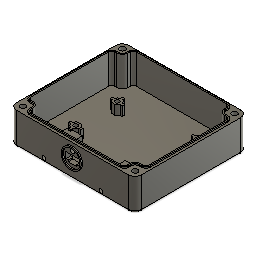
RPLIDAR Enclosure Base v7 (Autodesk Fusion 360 design; units mm, degrees)
Autodesk Fusion 360 part; units mm, degrees
sketch "Sketch1" plane through (0, 0, 0) normal (0, 1, 0) x (1, 0, 0)
  line L0 (6.35, 0) -> (110.49, 0)
  line L1 (116.84, 6.35) -> (116.84, 72.0491)
  line L2 (0, 72.0491) -> (0, 6.35)
  arc A0 (0, 6.35) -> (6.35, 0) centre (6.35, 6.35) ccw
  arc A1 (110.49, 0) -> (116.84, 6.35) centre (110.49, 6.35) ccw
  arc A2 (112.9511, 77.9028) -> (58.42, 88.9) centre (58.42, -51.7982) ccw
  arc A3 (58.42, 88.9) -> (3.8889, 77.9027) centre (58.42, -51.7979) ccw
  arc A4 (3.8889, 77.9027) -> (0, 72.0491) centre (6.35, 72.0491) ccw
  arc A5 (116.84, 72.0491) -> (112.9511, 77.9028) centre (110.49, 72.0491) ccw
  line L3 (2.286, 72.0491) -> (2.286, 6.35)
  arc A6 (2.286, 6.35) -> (6.35, 2.286) centre (6.35, 6.35) ccw
  line L4 (6.35, 2.286) -> (110.49, 2.286)
  arc A7 (110.49, 2.286) -> (114.554, 6.35) centre (110.49, 6.35) ccw
  line L5 (114.554, 6.35) -> (114.554, 72.0491)
  arc A8 (114.554, 72.0491) -> (112.0651, 75.7954) centre (110.49, 72.0491) ccw
  arc A9 (112.0651, 75.7954) -> (58.42, 86.614) centre (58.42, -51.7982) ccw
  arc A10 (58.42, 86.614) -> (4.7749, 75.7954) centre (58.42, -51.7979) ccw
  arc A11 (4.7749, 75.7954) -> (2.286, 72.0491) centre (6.35, 72.0491) ccw
  point P0 (116.84, 0)
  dimension "d1" = 116.84
  dimension "d3" = 6.35
  dimension "d4" = 6.35
  dimension "d5" = 6.35
  dimension "d6" = 6.35
  dimension "d7" = 2.286
  constraint horizontal L0
  constraint vertical L1
  constraint vertical L2
  constraint coincident origin L0
  constraint coincident origin L2
  constraint tangent L0 A0
  constraint tangent L2 A0
  constraint coincident P0 L0
  constraint coincident P0 L1
  constraint tangent L0 A1
  constraint tangent L1 A1
  constraint tangent A3 A4
  constraint tangent L2 A4
  constraint tangent A2 A5
  constraint tangent L1 A5
  measures "d1" distance of origin P0
  measures "d3" radius of A0
  measures "d4" radius of A1
  measures "d5" radius of A4
  measures "d6" radius of A5
mesh "Mesh1" [no effect]
sketch "Sketch2" plane through (0, 0, 0) normal (0, 1, 0) x (-1, 0, 0)
  line L0 (-23.4602, -26.5297) -> (-24.9674, -28.9918)
  line L1 (-24.9674, -28.9918) -> (-27.8532, -28.9176)
  line L2 (-27.8532, -28.9176) -> (-29.2318, -26.3814)
  line L3 (-29.2318, -26.3814) -> (-27.7247, -23.9193)
  line L4 (-27.7247, -23.9193) -> (-24.8389, -23.9934)
  line L5 (-24.8389, -23.9934) -> (-23.4602, -26.5297)
  circle A0 centre (-22.846, -46.4555) radius 15.9986
  circle A1 centre (-26.3276, -66.4551) radius 2.7647
  circle A2 centre (-26.3276, -26.456) radius 2.7647
  circle A3 centre (-96.3501, -74.4876) radius 2.7745
  circle A4 centre (-96.3712, -18.4353) radius 2.7744
sketch "Sketch3" plane through (0, 0, 0) normal (0, 1, 0) x (1, 0, 0)
  line L0 (13.5354, -5.4011) -> (100.9114, -5.4011)
  line L1 (115.3275, 9.026) -> (115.1243, 84.21)
  line L2 (100.9114, 98.6151) -> (13.5354, 98.6151)
  line L3 (-0.8807, 84.188) -> (-0.6775, 9.004)
  line L4 (104.9754, -1.3371) -> (104.9754, 0.887)
  line L5 (109.0394, 4.951) -> (111.2635, 4.951)
  line L6 (9.4714, -1.3371) -> (9.4714, 0.887)
  line L7 (5.4074, 4.951) -> (3.3865, 4.951)
  line L8 (104.9754, 94.5511) -> (104.9754, 92.327)
  line L9 (109.0394, 88.263) -> (111.0603, 88.263)
  line L10 (9.4714, 94.5511) -> (9.4714, 92.327)
  line L11 (5.4074, 88.263) -> (3.1833, 88.263)
  circle A0 centre (3.2484, 94.486) radius 2.9718
  circle A1 centre (111.1984, 94.486) radius 2.9718
  circle A2 centre (111.1984, -1.27) radius 2.9718
  circle A3 centre (3.2484, -1.27) radius 2.9718
  arc A4 (104.9754, 94.5511) -> (100.9114, 98.6151) centre (100.9114, 94.5511) ccw
  arc A5 (115.1243, 84.21) -> (111.0603, 88.263) centre (111.0603, 84.199) ccw
  arc A6 (104.9754, 92.327) -> (109.0394, 88.263) centre (109.0394, 92.327) ccw
  arc A7 (111.2635, 4.951) -> (115.3275, 9.026) centre (111.2635, 9.015) ccw
  arc A8 (100.9114, -5.4011) -> (104.9754, -1.3371) centre (100.9114, -1.3371) ccw
  arc A9 (109.0394, 4.951) -> (104.9754, 0.887) centre (109.0394, 0.887) ccw
  line L12 (3.4676, -7.7324) -> (111.1636, -7.7324)
  line L13 (117.5136, -1.3824) -> (117.5136, 94.1216)
  line L14 (111.1636, 100.4716) -> (3.4676, 100.4716)
  line L15 (-2.8824, 94.1216) -> (-2.8824, -1.3824)
  arc A10 (3.4676, 100.4716) -> (-2.8824, 94.1216) centre (3.4676, 94.1216) ccw
  arc A11 (117.5136, 94.1216) -> (111.1636, 100.4716) centre (111.1636, 94.1216) ccw
  arc A12 (111.1636, -7.7324) -> (117.5136, -1.3824) centre (111.1636, -1.3824) ccw
  arc A13 (-2.8824, -1.3824) -> (3.4676, -7.7324) centre (3.4676, -1.3824) ccw
  arc A14 (13.5354, 98.6151) -> (9.4714, 94.5511) centre (13.5354, 94.5511) ccw
  arc A15 (3.1833, 88.263) -> (-0.8807, 84.188) centre (3.1833, 84.199) ccw
  arc A16 (-0.6775, 9.004) -> (3.3865, 4.951) centre (3.3865, 9.015) ccw
  arc A17 (9.4714, -1.3371) -> (13.5354, -5.4011) centre (13.5354, -1.3371) ccw
  arc A18 (9.4714, 0.887) -> (5.4074, 4.951) centre (5.4074, 0.887) ccw
  arc A19 (5.4074, 88.263) -> (9.4714, 92.327) centre (5.4074, 92.327) ccw
  circle A20 centre (96.3501, 74.4876) radius 2.0193
  circle A21 centre (96.3712, 18.4353) radius 2.0193
  circle A22 centre (26.3276, 26.456) radius 2.0193
  circle A23 centre (26.3276, 66.4551) radius 2.0193
  arc A24 (27.2538, 62.498) -> (24.1187, 63.0438) centre (22.846, 46.4555) ccw
  arc A25 (24.1186, 29.8673) -> (27.2538, 30.413) centre (22.846, 46.4555) ccw
  line L16 (90.3811, 73.4716) -> (90.3811, 75.5036)
  line L17 (102.3191, 75.5036) -> (102.3191, 73.4716)
  line L18 (102.3191, 73.4716) -> (90.3811, 75.5036) construction
  line L19 (90.3811, 73.4716) -> (102.3191, 75.5036) construction
  line L20 (97.3661, 80.4566) -> (95.3341, 80.4566)
  line L21 (95.3341, 68.5186) -> (97.3661, 68.5186)
  line L22 (97.3661, 80.4566) -> (95.3341, 68.5186) construction
  line L23 (95.3341, 80.4566) -> (97.3661, 68.5186) construction
  line L24 (95.3341, 80.4566) -> (95.3341, 78.4226)
  line L25 (95.3341, 70.5527) -> (95.3341, 68.5186)
  line L26 (97.3661, 68.5186) -> (97.3661, 70.5527)
  line L27 (97.3661, 78.4226) -> (97.3661, 80.4566)
  arc A26 (97.3661, 70.5527) -> (100.2851, 73.4716) centre (96.3501, 74.4876) ccw
  arc A27 (100.2851, 75.5036) -> (97.3661, 78.4226) centre (96.3501, 74.4876) ccw
  line L28 (102.3191, 73.4716) -> (100.2851, 73.4716)
  line L29 (92.4152, 73.4716) -> (90.3811, 73.4716)
  arc A28 (95.3341, 78.4226) -> (92.4152, 75.5036) centre (96.3501, 74.4876) ccw
  arc A29 (92.4152, 73.4716) -> (95.3341, 70.5527) centre (96.3501, 74.4876) ccw
  line L30 (90.3811, 75.5036) -> (92.4152, 75.5036)
  line L31 (100.2851, 75.5036) -> (102.3191, 75.5036)
  line L32 (97.3872, 24.4043) -> (95.3552, 24.4043)
  line L33 (95.3552, 12.4663) -> (97.3872, 12.4663)
  line L34 (97.3872, 24.4043) -> (95.3552, 12.4663) construction
  line L35 (95.3552, 24.4043) -> (97.3872, 12.4663) construction
  line L36 (90.4022, 19.4513) -> (90.4022, 17.4193)
  line L37 (102.3402, 17.4193) -> (102.3402, 19.4513)
  line L38 (102.3402, 19.4513) -> (90.4022, 17.4193) construction
  line L39 (90.4022, 19.4513) -> (102.3402, 17.4193) construction
  line L40 (97.3872, 12.4663) -> (97.3872, 14.5004)
  line L41 (97.3872, 22.3703) -> (97.3872, 24.4043)
  line L42 (95.3552, 24.4043) -> (95.3552, 22.3703)
  line L43 (95.3552, 14.5004) -> (95.3552, 12.4663)
  arc A30 (97.3872, 14.5004) -> (100.3061, 17.4193) centre (96.3712, 18.4353) ccw
  arc A31 (100.3061, 19.4513) -> (97.3872, 22.3703) centre (96.3712, 18.4353) ccw
  line L44 (90.4022, 17.4193) -> (92.4362, 17.4193)
  line L45 (100.3061, 17.4193) -> (102.3402, 17.4193)
  arc A32 (95.3552, 22.3703) -> (92.4362, 19.4513) centre (96.3712, 18.4353) ccw
  arc A33 (92.4362, 17.4193) -> (95.3552, 14.5004) centre (96.3712, 18.4353) ccw
  line L46 (102.3402, 19.4513) -> (100.3061, 19.4513)
  line L47 (92.4362, 19.4513) -> (90.4022, 19.4513)
  line L48 (20.3586, 25.44) -> (20.3586, 27.472)
  line L49 (32.2966, 27.472) -> (32.2966, 25.44)
  line L50 (32.2966, 25.44) -> (20.3586, 27.472) construction
  line L51 (20.3586, 25.44) -> (32.2966, 27.472) construction
  line L52 (20.3586, 27.472) -> (22.3926, 27.472)
  line L53 (30.2625, 27.472) -> (32.2966, 27.472)
  arc A34 (30.2625, 27.472) -> (27.2538, 30.413) centre (26.3276, 26.456) ccw
  line L54 (32.2966, 25.44) -> (30.2625, 25.44)
  line L55 (22.3926, 25.44) -> (20.3586, 25.44)
  arc A35 (24.1186, 29.8673) -> (22.3926, 27.472) centre (26.3276, 26.456) ccw
  line L56 (27.3436, 20.487) -> (25.3116, 20.487)
  line L57 (27.3436, 22.5211) -> (27.3436, 20.487)
  line L58 (27.3436, 20.487) -> (25.3116, 32.425) construction
  line L59 (25.3116, 20.487) -> (27.3436, 32.425) construction
  arc A36 (22.3926, 25.44) -> (25.3116, 22.5211) centre (26.3276, 26.456) ccw
  arc A37 (27.3436, 22.5211) -> (30.2625, 25.44) centre (26.3276, 26.456) ccw
  line L60 (25.3116, 20.487) -> (25.3116, 22.5211)
  line L61 (20.3586, 67.4711) -> (20.3586, 65.4391)
  line L62 (32.2966, 65.4391) -> (32.2966, 67.4711)
  line L63 (32.2966, 67.4711) -> (20.3586, 65.4391) construction
  line L64 (20.3586, 67.4711) -> (32.2966, 65.4391) construction
  arc A38 (22.3926, 65.4391) -> (24.1187, 63.0438) centre (26.3276, 66.4551) ccw
  line L65 (32.2966, 67.4711) -> (30.2625, 67.4711)
  line L66 (22.3926, 67.4711) -> (20.3586, 67.4711)
  line L67 (20.3586, 65.4391) -> (22.3926, 65.4391)
  line L68 (30.2625, 65.4391) -> (32.2966, 65.4391)
  arc A39 (27.2538, 62.498) -> (30.2625, 65.4391) centre (26.3276, 66.4551) ccw
  line L69 (27.3436, 72.4241) -> (25.3116, 72.4241)
  line L70 (27.3436, 72.4241) -> (25.3116, 60.4861) construction
  line L71 (25.3116, 72.4241) -> (27.3436, 60.4861) construction
  arc A40 (30.2625, 67.4711) -> (27.3436, 70.39) centre (26.3276, 66.4551) ccw
  arc A41 (25.3116, 70.39) -> (22.3926, 67.4711) centre (26.3276, 66.4551) ccw
  line L72 (25.3116, 72.4241) -> (25.3116, 70.39)
  line L73 (27.3436, 70.39) -> (27.3436, 72.4241)
  line L74 (5.4074, 6.1702) -> (3.3865, 6.1702)
  arc A42 (0.5417, 9.0073) -> (3.3865, 6.1702) centre (3.3865, 9.015) ccw
  line L75 (0.3385, 84.1913) -> (0.5417, 9.0073)
  arc A43 (3.1833, 87.0438) -> (0.3385, 84.1913) centre (3.1833, 84.199) ccw
  line L76 (5.4074, 87.0438) -> (3.1833, 87.0438)
  arc A44 (5.4074, 87.0438) -> (10.6906, 92.327) centre (5.4074, 92.327) ccw
  line L77 (10.6906, 94.5511) -> (10.6906, 92.327)
  arc A45 (13.5354, 97.3959) -> (10.6906, 94.5511) centre (13.5354, 94.5511) ccw
  line L78 (100.9114, 97.3959) -> (13.5354, 97.3959)
  arc A46 (103.7562, 94.5511) -> (100.9114, 97.3959) centre (100.9114, 94.5511) ccw
  line L79 (103.7562, 94.5511) -> (103.7562, 92.327)
  arc A47 (103.7562, 92.327) -> (109.0394, 87.0438) centre (109.0394, 92.327) ccw
  line L80 (109.0394, 87.0438) -> (111.0603, 87.0438)
  arc A48 (113.9051, 84.2067) -> (111.0603, 87.0438) centre (111.0603, 84.199) ccw
  line L81 (114.1083, 9.0227) -> (113.9051, 84.2067)
  arc A49 (111.2635, 6.1702) -> (114.1083, 9.0227) centre (111.2635, 9.015) ccw
  line L82 (109.0394, 6.1702) -> (111.2635, 6.1702)
  arc A50 (109.0394, 6.1702) -> (103.7562, 0.887) centre (109.0394, 0.887) ccw
  line L83 (103.7562, -1.3371) -> (103.7562, 0.887)
  arc A51 (100.9114, -4.1819) -> (103.7562, -1.3371) centre (100.9114, -1.3371) ccw
  line L84 (13.5354, -4.1819) -> (100.9114, -4.1819)
  arc A52 (10.6906, -1.3371) -> (13.5354, -4.1819) centre (13.5354, -1.3371) ccw
  line L85 (10.6906, -1.3371) -> (10.6906, 0.887)
  arc A53 (10.6906, 0.887) -> (5.4074, 6.1702) centre (5.4074, 0.887) ccw
  line L86 (14.265, -3.1639) -> (101.4284, -3.1639)
  arc A54 (10.6906, -0.3368) -> (14.265, -3.1639) centre (14.265, 0.5093) ccw
  arc A55 (101.4284, -3.1639) -> (103.7562, -1.3426) centre (101.4284, -0.7657) ccw
  line L87 (23.0256, -7.7324) -> (36.7416, -7.7324)
  line L88 (36.7416, -7.7324) -> (36.7416, 22.4936)
  line L89 (36.7416, 22.4936) -> (23.0256, 22.4936)
  line L90 (23.0256, 22.4936) -> (23.0256, -7.7324)
  line L91 (91.6056, -7.7324) -> (77.8896, -7.7324)
  line L92 (77.8896, -7.7324) -> (77.8896, 22.4936)
  line L93 (77.8896, 22.4936) -> (91.6056, 22.4936)
  line L94 (91.6056, 22.4936) -> (91.6056, -7.7324)
  line L95 (26.0736, 11.8256) -> (33.6936, 11.8256)
  line L96 (33.6936, 11.8256) -> (33.6936, -2.9064)
  line L97 (33.6936, -2.9064) -> (26.0736, -2.9064)
  line L98 (26.0736, -2.9064) -> (26.0736, 11.8256)
  line L99 (80.9376, 11.8256) -> (88.5576, 11.8256)
  line L100 (88.5576, 11.8256) -> (88.5576, -2.9064)
  line L101 (88.5576, -2.9064) -> (80.9376, -2.9064)
  line L102 (80.9376, -2.9064) -> (80.9376, 11.8256)
  point P0 (-2.8824, -7.7324)
  point P1 (117.5136, -7.7324)
  point P2 (-2.8824, 100.4716)
  point P3 (26.3276, 66.4551)
  point P4 (26.3276, 26.456)
  point P5 (96.3712, 18.4353)
  point P6 (96.3501, 74.4876)
  point P7 (22.846, 46.4555)
  point P8 (96.3501, 74.4876)
  point P9 (96.3501, 74.4876)
  point P10 (96.3712, 18.4353)
  point P11 (96.3712, 18.4353)
  point P12 (26.3276, 26.456)
  point P13 (26.3276, 26.456)
  point P14 (26.3276, 66.4551)
  point P15 (26.3276, 66.4551)
  dimension "d19" = 5.9436
  dimension "d20" = 5.9436
  dimension "d21" = 5.9436
  dimension "d22" = 5.9436
  dimension "d23" = 4.064
  dimension "d24" = 4.064
  dimension "d26" = 4.064
  dimension "d27" = 4.064
  dimension "d28" = 4.064
  dimension "d29" = 4.064
  dimension "d31" = 120.396
  dimension "d32" = 108.204
  dimension "d33" = 6.35
  dimension "d34" = 6.35
  dimension "d35" = 6.35
  dimension "d36" = 6.35
  dimension "d37" = 4.064
  dimension "d38" = 4.064
  dimension "d39" = 4.064
  dimension "d40" = 4.064
  dimension "d41" = 4.064
  dimension "d42" = 4.064
  dimension "d43" = 8.128
  dimension "d44" = 8.128
  dimension "d45" = 8.128
  dimension "d46" = 8.128
  dimension "d47" = 4.0386
  dimension "d48" = 4.0386
  dimension "d49" = 4.0386
  dimension "d50" = 4.0386
  dimension "d52" = 33.274
  dimension "d53" = 11.938
  dimension "d54" = 2.032
  dimension "d55" = 2.032
  dimension "d56" = 11.938
  dimension "d57" = 11.938
  dimension "d58" = 2.032
  dimension "d59" = 11.938
  dimension "d60" = 2.032
  dimension "d61" = 11.938
  dimension "d62" = 2.032
  dimension "d63" = 2.032
  dimension "d64" = 11.938
  dimension "d65" = 11.938
  dimension "d66" = 2.032
  dimension "d67" = 2.032
  dimension "d68" = 11.938
  dimension "d71" = 1.2192
  dimension "d121" = 5.9856
  dimension "d122" = 6.1308
  dimension "d124" = 12.2086
  dimension "d125" = 12.2086
  dimension "d126" = 5.9856
  dimension "d127" = 6.3152
  dimension "d129" = 70.0436
  dimension "d130" = 56.0523
  dimension "d131" = 34.1884
  dimension "d132" = 2.1861
  dimension "d133" = 2.3893
  dimension "d134" = 6.3152
  dimension "d135" = 2.2049
  dimension "d136" = 2.0017
  dimension "d137" = 6.1308
  dimension "d138" = 12.3538
  dimension "d139" = 12.3538
  dimension "d140" = 12.5382
  dimension "d141" = 12.5382
  dimension "d186" = 1.8565
  dimension "d187" = 6.4624
  dimension "d188" = 6.4624
  dimension "d189" = 1.018
  dimension "d190" = 12.6834
  dimension "d191" = 12.6834
  dimension "d192" = 2.3313
  dimension "d198" = 29.21
  dimension "d214" = 13.716
  dimension "d215" = 30.226
  dimension "d216" = 13.716
  dimension "d217" = 30.226
  dimension "d218" = 25.908
  dimension "d219" = 25.908
  dimension "d220" = 7.62
  dimension "d221" = 14.732
  dimension "d222" = 3.048
  dimension "d223" = 4.826
  dimension "d224" = 7.62
  dimension "d225" = 14.732
  dimension "d226" = 4.826
  dimension "d227" = 3.048
  constraint vertical L4
  constraint horizontal L5
  constraint vertical L6
  constraint horizontal L7
  constraint vertical L8
  constraint horizontal L9
  constraint vertical L10
  constraint horizontal L11
  constraint tangent L8 A4
  constraint tangent L2 A4
  constraint tangent L1 A5
  constraint tangent L9 A5
  constraint tangent L8 A6
  constraint tangent L9 A6
  constraint tangent L5 A7
  constraint tangent L1 A7
  constraint tangent L4 A8
  constraint tangent L0 A8
  constraint tangent L4 A9
  constraint tangent L5 A9
  constraint horizontal L12
  constraint vertical L13
  constraint horizontal L14
  constraint vertical L15
  constraint coincident P2 L14
  constraint coincident P2 L15
  constraint tangent L14 A10
  constraint tangent L15 A10
  constraint tangent L13 A11
  constraint tangent L14 A11
  constraint coincident P1 L12
  constraint coincident P1 L13
  constraint tangent L12 A12
  constraint tangent L13 A12
  constraint coincident P0 L12
  constraint coincident P0 L15
  constraint tangent L12 A13
  constraint tangent L15 A13
  constraint tangent L10 A14
  constraint tangent L2 A14
  constraint tangent L11 A15
  constraint tangent L3 A15
  constraint tangent L7 A16
  constraint tangent L3 A16
  constraint tangent L6 A17
  constraint tangent L0 A17
  constraint tangent L6 A18
  constraint tangent L7 A18
  constraint tangent L10 A19
  constraint tangent L11 A19
  constraint coincident P15 P14
  constraint coincident P13 P12
  constraint coincident P11 P10
  constraint coincident P9 P8
  constraint concentric A20 A28
  constraint concentric A21 A32
  constraint concentric A22 A35
  constraint concentric A23 A39
  constraint coincident P7 A24.centre
  constraint coincident A25.start A24
  constraint concentric A24 A25
  constraint perpendicular L16 L28
  constraint parallel L28 L30
  constraint parallel L16 L17
  constraint horizontal L28
  constraint coincident L18 P9
  constraint coincident L19 P9
  constraint perpendicular L20 L24
  constraint parallel L20 L21
  constraint parallel L24 L26
  constraint horizontal L20
  constraint coincident L22 P9
  constraint coincident L23 P9
  constraint coincident L27.start L26
  constraint collinear L24 L25
  constraint coincident L26.end A28
  constraint concentric A26 A28
  constraint concentric A26 A27
  constraint coincident A27.start L30
  constraint coincident L29.start A28
  constraint concentric A28 A29
  constraint collinear L30 L31
  constraint perpendicular L32 L42
  constraint parallel L32 L33
  constraint parallel L40 L42
  constraint horizontal L32
  constraint coincident L34 P11
  constraint coincident L35 P11
  constraint perpendicular L36 L46
  constraint parallel L44 L46
  constraint parallel L36 L37
  constraint horizontal L46
  constraint coincident L38 P11
  constraint coincident L39 P11
  constraint coincident L41.start L40
  constraint collinear L40 L41
  constraint coincident L40.end A32
  constraint collinear L42 L43
  constraint concentric A30 A32
  constraint coincident A30.end L44
  constraint concentric A30 A31
  constraint collinear L44 L45
  constraint coincident L44.end A32
  constraint concentric A32 A33
  constraint coincident A32.end L46
  constraint collinear L46 L47
  constraint perpendicular L48 L54
  constraint parallel L52 L54
  constraint parallel L48 L49
  constraint horizontal L54
  constraint coincident L50 P13
  constraint coincident L51 P13
  constraint collinear L52 L53
  constraint coincident L53.start A35
  constraint concentric A34 A35
  constraint collinear L54 L55
  constraint coincident L55.start A35
  constraint concentric A35 A36
  constraint perpendicular L56 L60
  constraint parallel L57 L60
  constraint horizontal L56
  constraint coincident L58 P13
  constraint coincident L59 P13
  constraint concentric A36 A37
  constraint perpendicular L61 L65
  constraint parallel L65 L67
  constraint parallel L61 L62
  constraint horizontal L65
  constraint coincident L63 P15
  constraint coincident L64 P15
  constraint concentric A38 A39
  constraint coincident L66.start L65
  constraint collinear L65 L66
  constraint coincident L65.end A39
  constraint collinear L67 L68
  constraint concentric A39 A40
  constraint perpendicular L69 L72
  constraint horizontal L69
  constraint coincident L70 P15
  constraint coincident L71 P15
  constraint concentric A40 A41
  constraint coincident L85 A54.start
  constraint tangent L86 A54
  constraint coincident L83 A55.end
  constraint tangent L86 A55
  constraint horizontal L87
  constraint vertical L88
  constraint horizontal L89
  constraint vertical L90
  constraint coincident L12 L87.start
  constraint horizontal L91
  constraint vertical L92
  constraint horizontal L93
  constraint vertical L94
  constraint coincident L12 L91.start
  constraint horizontal L95
  constraint vertical L96
  constraint horizontal L97
  constraint vertical L98
  constraint horizontal L99
  constraint vertical L100
  constraint horizontal L101
  constraint vertical L102
  measures "d19" diameter of A0
  measures "d20" diameter of A1
  measures "d21" diameter of A2
  measures "d22" diameter of A3
  measures "d23" radius of A4
  measures "d24" radius of A5
  measures "d26" radius of A6
  measures "d27" radius of A7
  measures "d28" radius of A8
  measures "d29" radius of A9
  measures "d31" distance of P0 P1
  measures "d32" distance of P0 P2
  measures "d33" radius of A10
  measures "d34" radius of A11
  measures "d35" radius of A12
  measures "d36" radius of A13
  measures "d37" radius of A14
  measures "d38" radius of A15
  measures "d39" radius of A16
  measures "d40" radius of A17
  measures "d41" radius of A18
  measures "d42" radius of A19
  measures "d43" diameter of A39
  measures "d44" diameter of A35
  measures "d45" diameter of A32
  measures "d46" diameter of A28
  measures "d47" diameter of A20
  measures "d48" diameter of A21
  measures "d49" diameter of A22
  measures "d50" diameter of A23
  measures "d52" diameter of A24
  measures "d53" distance of L16.end L17.start
  measures "d54" distance of L16.start L16.end
  measures "d55" distance of L21.start L21.end
  measures "d56" distance of L20.end L21.start
  measures "d57" distance of L32.end L33.start
  measures "d58" distance of L33.start L33.end
  measures "d59" distance of L36.end L37.start
  measures "d60" distance of L36.start L36.end
  measures "d61" distance of L48.end L49.start
  measures "d62" distance of L48.start L48.end
  measures "d63" distance of L58.end L59.end
  measures "d64" distance of L56.end L58.end
  measures "d65" distance of L61.end L62.start
  measures "d66" distance of L61.start L61.end
  measures "d67" distance of L70.end L71.end
  measures "d68" distance of L69.end L70.end
  measures "d121" vertical distance of A0.centre L14.end
  measures "d122" horizontal distance of A0.centre L15.start
  measures "d124" distance of L11 L14
  measures "d125" distance of L9 L14
  measures "d126" vertical distance of A1.centre L14.start
  measures "d127" horizontal distance of A1.centre L13.end
  measures "d129" horizontal distance of P11 P13
  measures "d130" vertical distance of P9 P11
  measures "d131" distance of L12 P13
  measures "d132" distance of L1.start L13
  measures "d133" distance of L1.end L13
  measures "d134" horizontal distance of A2.centre L13.start
  measures "d135" distance of L15 L3.end
  measures "d136" distance of L15 L3.start
  measures "d137" horizontal distance of A3.centre L15.end
  measures "d138" distance of L6 L15.end
  measures "d139" distance of L10 L15
  measures "d140" distance of L4 L13
  measures "d141" distance of L8 L13
  measures "d186" distance of L2 L14
  measures "d187" distance of A3.centre L12
  measures "d188" distance of A2.centre L12
  measures "d189" distance of L84 L86
  measures "d190" distance of L7 L12
  measures "d191" distance of L5 L12
  measures "d192" distance of L0 L12
  measures "d198" distance of L15 P13
  measures "d214" distance of L87.start L87.end
  measures "d215" distance of L87.start L89.end
  measures "d216" distance of L91.start L91.end
  measures "d217" distance of L91.start L93.end
  measures "d218" distance of L13 L94
  measures "d219" distance of L15 L90
  measures "d220" distance of L95.start L95.end
  measures "d221" distance of L95.start L97.end
  measures "d222" distance of L90 L98
  measures "d223" distance of L12 L97
  measures "d224" distance of L99.start L99.end
  measures "d225" distance of L99.start L101.end
  measures "d226" distance of L12 L101
  measures "d227" distance of L92 L102
extrude "Extrude11" add sketch "Sketch3" along normal blind 3.048 contours L84 L86 L88 L90 | L84 A52 L85 L86 A54 L90 | L84 L86 L88 L92 | L56 L57 L60 L86 L88 L89 L90 | A25 L32 L33 L37 L40 L41 L42 L43 A30 A31 L44 L45 A32 A33 L46 L47 L48 L49 L52 L53 A34 L54 L55 A35 L57 A36 A37 L60 L74 A42 L75 A43 L76 A44 L77 A45 L78 A46 L79 A47 L80 A48 L81 A49 L82 A50 L83 A51 L85 A53 L86 A54 A55 L88 L89 L90 L92 L93 L94 | L84 L86 L92 L94 | A51 L84 L86 A55 L94 | L36 L44 L47 L86 L92 L93 L94 | L95 L96 L97 L98 | L99 L100 L101 L102 makes body 1
extrude "Extrude12" add sketch "Sketch3" along normal blind 31.75 separate body contours L0 L1 L2 L3 L4 L5 L6 L7 L8 L9 L10 L11 A4 A5 A6 A7 A8 A9 A14 A15 A16 A17 A18 A19 L74 A42 L75 A43 L76 A44 L77 A45 L78 A46 L79 A47 L80 A48 L81 A49 L82 A50 L83 A51 L84 A52 L85 A53 L90 L94 | L0 L84 L88 L90 | L0 L84 L88 L92 | L0 L84 L92 L94 makes body 2
extrude "Extrude13" add sketch "Sketch3" along normal blind 30.48 contours L0 L1 L2 L3 L4 L5 L6 L7 L8 L9 L10 L11 A4 A5 A6 A7 A8 A9 L12 L13 L14 L15 A10 A11 A12 A13 A14 A15 A16 A17 A18 A19 L90 L94 | L0 L12 L87 L88 L90 | L0 L12 L88 L92 | L0 L12 L91 L92 L94 | A0 | A1 | A2 | A3 bodies 2
extrude "Extrude14" add sketch "Sketch3" along normal blind 12.192 contours L56 L57 L60 L89 | A25 L48 L49 L52 L53 A34 L54 L55 A35 L57 A36 A37 L60 L89 | L32 L33 L37 L40 L41 L42 L43 A30 A31 L44 L45 A32 A33 L46 L47 L94 | L36 L44 L47 L94 | A20 | A21 | A22 | A23 | A24 L61 L62 A38 L65 L66 L67 L68 A39 L69 A40 A41 L72 L73 | L16 L17 L20 L21 L24 L25 L26 L27 A26 A27 L28 L29 A28 A29 L30 L31 bodies 1
sketch "Sketch7" plane through (0, 12.192, 0) normal (0, 1, 0) x (-1, 0, 0)
  line L0 (-92.4362, -19.4513) -> (-90.4022, -19.4513)
  line L1 (-90.4022, -19.4513) -> (-90.4022, -17.4193)
  line L2 (-90.4022, -17.4193) -> (-92.4362, -17.4193)
  arc A0 (-92.4362, -17.4193) -> (-95.3552, -14.5004) centre (-96.3712, -18.4353) ccw
  line L3 (-95.3552, -14.5004) -> (-95.3552, -12.4663)
  line L4 (-95.3552, -12.4663) -> (-97.3872, -12.4663)
  line L5 (-97.3872, -12.4663) -> (-97.3872, -14.5004)
  arc A1 (-97.3872, -14.5004) -> (-100.3061, -17.4193) centre (-96.3712, -18.4353) ccw
  line L6 (-100.3061, -17.4193) -> (-102.3402, -17.4193)
  line L7 (-102.3402, -17.4193) -> (-102.3402, -19.4513)
  line L8 (-102.3402, -19.4513) -> (-100.3061, -19.4513)
  arc A2 (-100.3061, -19.4513) -> (-97.3872, -22.3703) centre (-96.3712, -18.4353) ccw
  line L9 (-97.3872, -22.3703) -> (-97.3872, -24.4043)
  line L10 (-97.3872, -24.4043) -> (-95.3552, -24.4043)
  line L11 (-95.3552, -24.4043) -> (-95.3552, -22.3703)
  arc A3 (-95.3552, -22.3703) -> (-92.4362, -19.4513) centre (-96.3712, -18.4353) ccw
  circle A4 centre (-96.3712, -18.4353) radius 2.0193
  dimension "d150" = 4.0386
  constraint concentric A0 A4
  measures "d150" diameter of A4
extrude "Extrude15" cut sketch "Sketch7" against normal blind 6.35 contours A4 bodies 1
draft "Draft9" angle 2.37 neutral plane through (0, 12.192, 0) pull (0, 1, 0) 1 faces at (96.4215, 7.9587, -16.4166) on bodies 1
sketch "Sketch8" plane through (0, 12.192, 0) normal (0, 1, 0) x (-1, 0, 0)
  arc A0 (-27.3436, -22.5211) -> (-30.2625, -25.44) centre (-26.3276, -26.456) ccw
  line L0 (-30.2625, -25.44) -> (-32.2966, -25.44)
  line L1 (-32.2966, -25.44) -> (-32.2966, -27.472)
  line L2 (-32.2966, -27.472) -> (-30.2625, -27.472)
  arc A1 (-30.2625, -27.472) -> (-27.2538, -30.413) centre (-26.3276, -26.456) ccw
  arc A2 (-24.1186, -29.8673) -> (-27.2538, -30.413) centre (-22.846, -46.4555) ccw
  arc A3 (-24.1186, -29.8673) -> (-22.3926, -27.472) centre (-26.3276, -26.456) ccw
  line L3 (-22.3926, -27.472) -> (-20.3586, -27.472)
  line L4 (-20.3586, -27.472) -> (-20.3586, -25.44)
  line L5 (-20.3586, -25.44) -> (-22.3926, -25.44)
  arc A4 (-22.3926, -25.44) -> (-25.3116, -22.5211) centre (-26.3276, -26.456) ccw
  line L6 (-25.3116, -22.5211) -> (-25.3116, -20.487)
  line L7 (-25.3116, -20.487) -> (-27.3436, -20.487)
  line L8 (-27.3436, -20.487) -> (-27.3436, -22.5211)
  circle A5 centre (-26.3276, -26.456) radius 2.0193
  circle A6 centre (-26.3276, -66.4551) radius 2.0193
  circle A7 centre (-96.3501, -74.4876) radius 2.0193
  point P0 (-26.3276, -66.4551)
  point P1 (-96.3501, -74.4876)
  constraint concentric A0 A5
  constraint coincident P0 A6.centre
  constraint coincident P1 A7.centre
extrude "Extrude16" cut sketch "Sketch8" against normal blind 6.35 contours A5 | A6 | A7 bodies 1
draft "Draft10" angle 2.37 neutral plane through (0, 12.192, 0) pull (0, 1, 0) 1 faces at (24.3183, 7.9587, -66.6561) on bodies 1
draft "Draft11" angle 2.37 neutral plane through (0, 12.192, 0) pull (0, 1, 0) 1 faces at (94.9402, 7.9587, -73.0421) on bodies 1
draft "Draft12" angle 2.37 neutral plane through (0, 12.192, 0) pull (0, 1, 0) 1 faces at (24.3183, 7.9587, -26.6571) on bodies 1
sketch "Sketch9" plane through (0, 30.48, 0) normal (0, 1, 0) x (-1, 0, 0)
  arc A0 (-3.1833, -88.263) -> (0.8807, -84.188) centre (-3.1833, -84.199) ccw
  line L0 (-3.1833, -88.263) -> (-5.4074, -88.263)
  arc A1 (-5.4074, -88.263) -> (-9.4714, -92.327) centre (-5.4074, -92.327) ccw
  line L1 (-9.4714, -92.327) -> (-9.4714, -94.5511)
  arc A2 (-13.5354, -98.6151) -> (-9.4714, -94.5511) centre (-13.5354, -94.5511) ccw
  line L2 (-13.5354, -98.6151) -> (-100.9114, -98.6151)
  arc A3 (-104.9754, -94.5511) -> (-100.9114, -98.6151) centre (-100.9114, -94.5511) ccw
  line L3 (-104.9754, -94.5511) -> (-104.9754, -92.327)
  arc A4 (-104.9754, -92.327) -> (-109.0394, -88.263) centre (-109.0394, -92.327) ccw
  line L4 (-109.0394, -88.263) -> (-111.0603, -88.263)
  arc A5 (-115.1243, -84.21) -> (-111.0603, -88.263) centre (-111.0603, -84.199) ccw
  line L5 (-115.1243, -84.21) -> (-115.3275, -9.026)
  arc A6 (-111.2635, -4.951) -> (-115.3275, -9.026) centre (-111.2635, -9.015) ccw
  line L6 (-111.2635, -4.951) -> (-109.0394, -4.951)
  arc A7 (-109.0394, -4.951) -> (-104.9754, -0.887) centre (-109.0394, -0.887) ccw
  line L7 (-104.9754, -0.887) -> (-104.9754, 1.3371)
  arc A8 (-100.9114, 5.4011) -> (-104.9754, 1.3371) centre (-100.9114, 1.3371) ccw
  line L8 (-100.9114, 5.4011) -> (-13.5354, 5.4011)
  arc A9 (-9.4714, 1.3371) -> (-13.5354, 5.4011) centre (-13.5354, 1.3371) ccw
  line L9 (-9.4714, 1.3371) -> (-9.4714, -0.887)
  arc A10 (-9.4714, -0.887) -> (-5.4074, -4.951) centre (-5.4074, -0.887) ccw
  line L10 (-5.4074, -4.951) -> (-3.3865, -4.951)
  arc A11 (0.6775, -9.004) -> (-3.3865, -4.951) centre (-3.3865, -9.015) ccw
  line L11 (0.6775, -9.004) -> (0.8807, -84.188)
  arc A12 (2.8824, 1.3824) -> (-3.4676, 7.7324) centre (-3.4676, 1.3824) ccw
  line L12 (-3.4676, 7.7324) -> (-111.1636, 7.7324)
  arc A13 (-111.1636, 7.7324) -> (-117.5136, 1.3824) centre (-111.1636, 1.3824) ccw
  line L13 (-117.5136, 1.3824) -> (-117.5136, -94.1216)
  arc A14 (-117.5136, -94.1216) -> (-111.1636, -100.4716) centre (-111.1636, -94.1216) ccw
  line L14 (-111.1636, -100.4716) -> (-3.4676, -100.4716)
  arc A15 (-3.4676, -100.4716) -> (2.8824, -94.1216) centre (-3.4676, -94.1216) ccw
  line L15 (2.8824, -94.1216) -> (2.8824, 1.3824)
  circle A16 centre (-3.2484, -94.486) radius 2.6162
  circle A17 centre (-111.1984, -94.486) radius 2.6162
  circle A18 centre (-111.1984, 1.27) radius 2.6162
  circle A19 centre (-3.2484, 1.27) radius 2.6162
  point P0 (-3.2484, -94.486)
  point P1 (-111.1984, -94.486)
  point P2 (-111.1984, 1.27)
  point P3 (-3.2484, 1.27)
  dimension "d246" = 5.2324
  dimension "d247" = 5.2324
  dimension "d248" = 5.2324
  dimension "d249" = 5.2324
  constraint coincident P0 A16.centre
  constraint coincident P1 A17.centre
  constraint coincident P2 A18.centre
  constraint coincident P3 A19.centre
  measures "d246" diameter of A16
  measures "d247" diameter of A17
  measures "d248" diameter of A19
  measures "d249" diameter of A18
extrude "Extrude17" cut sketch "Sketch9" against normal blind 6.604 contours A16 | A17 | A18 | A19 bodies 2
draft "Draft13" angle 2.4 neutral plane through (0, 30.48, 0) pull (0, 1, 0) 1 faces at (110.8731, 26.0773, -91.8901) on bodies 2
draft "Draft14" angle 2.4 neutral plane through (0, 30.48, 0) pull (0, 1, 0) 1 faces at (110.8731, 26.0773, 3.8659) on bodies 2
draft "Draft15" angle 2.4 neutral plane through (0, 30.48, 0) pull (0, 1, 0) 1 faces at (0.6354, 26.0773, 1.1396) on bodies 2
draft "Draft16" angle 2.4 neutral plane through (0, 30.48, 0) pull (0, 1, 0) 1 faces at (4.6678, 26.0773, -92.2883) on bodies 2
sketch "Sketch10" plane through (0, 0, 7.7324) normal (0, 0, 1) x (1, 0, 0)
  line L0 (3.4676, 0) -> (111.1636, 0)
  line L1 (111.1636, 0) -> (111.1636, 30.48)
  line L2 (111.1636, 30.48) -> (3.4676, 30.48)
  line L3 (3.4676, 30.48) -> (3.4676, 0)
  circle A0 centre (57.3156, 17.78) radius 8.509
  line L4 (-2.8824, 0) -> (-2.8824, 30.48)
  line L5 (3.4676, 0) -> (111.1636, 0)
  line L6 (117.5136, 0) -> (117.5136, 30.48)
  circle A1 centre (57.3156, 17.78) radius 9.7282
  line L7 (50.9656, 19.812) -> (63.6656, 19.812)
  line L8 (63.6656, 19.812) -> (63.6656, 13.97)
  line L9 (63.6656, 13.97) -> (50.9656, 13.97)
  line L10 (50.9656, 13.97) -> (50.9656, 19.812)
  circle A2 centre (57.3156, 23.114) radius 1.8796
  line L11 (61.3796, 13.97) -> (53.2516, 13.97)
  line L12 (53.2516, 13.97) -> (53.2516, 12.446)
  line L13 (53.2516, 12.446) -> (61.3796, 12.446)
  line L14 (61.3796, 12.446) -> (61.3796, 13.97)
  dimension "d173" = 17.018
  dimension "d174" = 60.198
  dimension "d175" = 17.78
  dimension "d199" = 1.2192
  dimension "d201" = 12.7
  dimension "d202" = 5.842
  dimension "d203" = 6.35
  dimension "d204" = 2.032
  dimension "d205" = 3.7592
  dimension "d206" = 5.334
  dimension "d241" = 8.128
  dimension "d242" = 1.524
  dimension "d243" = 2.286
  constraint horizontal L7
  constraint vertical L8
  constraint horizontal L9
  constraint vertical L10
  constraint horizontal L11
  constraint vertical L12
  constraint horizontal L13
  constraint vertical L14
  constraint coincident L9 L11.start
  measures "d173" diameter of A0
  measures "d174" distance of A0.centre L4
  measures "d175" distance of A0.centre L5
  measures "d201" distance of L7.start L7.end
  measures "d202" distance of L7.start L9.end
  measures "d203" distance of A0.centre L8
  measures "d204" distance of A0.centre L7
  measures "d205" diameter of A2
  measures "d206" distance of A0.centre A2.centre
  measures "d241" distance of L11.start L11.end
  measures "d242" distance of L11.start L13.end
  measures "d243" distance of L8 L14
fillet "Fillet2" radius 1.6002 8 edges at (117.5136, 0, -46.3696) (115.6537, 0, -98.6117) (57.3156, 0, -100.4716) (-1.0226, 0, -98.6117) (-2.8824, 0, -46.3696) (-1.0226, 0, 5.8725) (57.3156, 0, 7.7324) (115.6537, 0, 5.8725) on bodies 2
extrude "Extrude20" add sketch "Sketch3" along normal blind 30.48 contours L84 L86 L88 L90 | L84 A52 L85 L86 A54 L90 | L84 L86 L88 L92 | L84 L86 L92 L94 | A51 L84 L86 A55 L94 bodies 1 2
extrude "Extrude22" cut sketch "Sketch10" against normal blind 5.08 contours L7 L8 L9 L10 L11 bodies 1
extrude "Extrude23" cut sketch "Sketch10" against normal blind 5.08 contours A2 bodies 1
extrude "Extrude24" add sketch "Sketch10" along normal blind 1.27 contours A1 bodies 1
extrude "Extrude25" add sketch "Sketch3" along normal blind 10.668 contours L56 L57 L60 L86 L88 L89 L90 | L36 L44 L47 L86 L92 L93 L94 | L56 L57 L60 L89 | L95 L96 L97 L98 | L99 L100 L101 L102 bodies 1
extrude "Extrude26" cut sketch "Sketch3" along normal blind 7.62 contours L95 L96 L97 L98 | L99 L100 L101 L102 bodies 1
chamfer "Chamfer1" distance 7.62 angle 45 2 edges at (84.7476, 0, -11.8256) (29.8836, 0, -11.8256) on bodies 1
fillet "Fillet3" radius 3.81 2 edges at (80.9376, 7.62, -4.4596) (88.5576, 7.62, -4.4596) on bodies 1
fillet "Fillet4" radius 3.81 2 edges at (33.6936, 7.62, -4.4596) (26.0736, 7.62, -4.4596) on bodies 1
sketch "Sketch14" plane through (0, 0, 2.9064) normal (0, 0, -1) x (-1, 0, 0)
  arc A0 (-80.9376, 3.81) -> (-88.5576, 3.81) centre (-84.7476, 3.81) ccw
  line L0 (-88.5576, 3.81) -> (-88.5576, 0)
  line L1 (-88.5576, 0) -> (-80.9376, 0)
  line L2 (-80.9376, 0) -> (-80.9376, 3.81)
  circle A1 centre (-84.7476, 3.81) radius 1.8923
  line L3 (-111.1636, 0) -> (-3.4676, 0)
  dimension "d235" = 3.7846
  dimension "d236" = 3.81
  measures "d235" diameter of A1
  measures "d236" distance of A0.centre L3
sketch "Sketch15" plane through (0, 0, 2.9064) normal (0, 0, -1) x (-1, 0, 0)
  arc A0 (-26.0736, 3.81) -> (-33.6936, 3.81) centre (-29.8836, 3.81) ccw
  line L0 (-33.6936, 3.81) -> (-33.6936, 0)
  line L1 (-33.6936, 0) -> (-26.0736, 0)
  line L2 (-26.0736, 0) -> (-26.0736, 3.81)
  circle A1 centre (-29.8836, 3.81) radius 1.8923
  line L3 (-111.1636, 0) -> (-3.4676, 0)
  dimension "d237" = 3.7846
  dimension "d238" = 3.81
  measures "d237" diameter of A1
  measures "d238" distance of A0.centre L3
extrude "Extrude27" cut sketch "Sketch15" sketch "Sketch14" against normal blind 5.08 contours A1 of sketch 2 contours A1 bodies 1
extrude "Extrude28" cut sketch "Sketch10" against normal blind 5.08 contours L9 L11 L12 L13 L14 bodies 1
extrude "Extrude1" add sketch "Sketch3" along normal blind 3.048 separate body contours L56 L57 L60 L86 L88 L89 L90 | A25 L32 L33 L37 L40 L41 L42 L43 A30 A31 L44 L45 A32 A33 L46 L47 L48 L49 L52 L53 A34 L54 L55 A35 L57 A36 A37 L60 L74 A42 L75 A43 L76 A44 L77 A45 L78 A46 L79 A47 L80 A48 L81 A49 L82 A50 L83 A51 L85 A53 L86 A54 A55 L88 L89 L90 L92 L93 L94 | L36 L44 L47 L86 L92 L93 L94 | L95 L96 L97 L98 | L99 L100 L101 L102 makes body 3
extrude "Extrude2" add sketch "Sketch3" along normal blind 7.4422 separate body contours A23 makes body 4
extrude "Extrude3" add sketch "Sketch3" along normal blind 7.4422 separate body contours A20 makes body 5
extrude "Extrude4" add sketch "Sketch3" along normal blind 7.4422 separate body contours A21 makes body 6
extrude "Extrude5" add sketch "Sketch3" along normal blind 7.4422 separate body contours A22 makes body 7
extrude "Extrude6" add sketch "Sketch3" along normal blind 12.954 contours L56 L57 L60 L89 | A25 L48 L49 L52 L53 A34 L54 L55 A35 L57 A36 A37 L60 L89 | L32 L33 L37 L40 L41 L42 L43 A30 A31 L44 L45 A32 A33 L46 L47 L94 | L36 L44 L47 L94 | A24 L61 L62 A38 L65 L66 L67 L68 A39 L69 A40 A41 L72 L73 | L16 L17 L20 L21 L24 L25 L26 L27 A26 A27 L28 L29 A28 A29 L30 L31 bodies 3 4 5 6 7
extrude "Extrude7" add sketch "Sketch3" along normal blind 23.3426 separate body contours A0 | A1 | A2 | A3 makes body 8 at (111.1243, 15.5617, -97.4568) makes body 9 at (111.1243, 15.5617, -1.7009) makes body 10 at (0.6385, 15.5617, -95.9072) makes body 11 at (6.2165, 15.5617, 1.4181)
extrude "Extrude8" add sketch "Sketch3" along normal blind 31.242 contours L0 L1 L2 L3 L4 L5 L6 L7 L8 L9 L10 L11 A4 A5 A6 A7 A8 A9 L12 L13 L14 L15 A10 A11 A12 A13 A14 A15 A16 A17 A18 A19 L90 L94 | L0 L12 L87 L88 L90 | L0 L12 L88 L92 | L84 L86 L88 L90 | L84 A52 L85 L86 A54 L90 | L0 L12 L91 L92 L94 | L84 L86 L88 L92 | L84 L86 L92 L94 | A51 L84 L86 A55 L94 bodies 3 8 9 10 11
extrude "Extrude9" add sketch "Sketch3" along normal blind 32.512 contours L0 L1 L2 L3 L4 L5 L6 L7 L8 L9 L10 L11 A4 A5 A6 A7 A8 A9 A14 A15 A16 A17 A18 A19 L74 A42 L75 A43 L76 A44 L77 A45 L78 A46 L79 A47 L80 A48 L81 A49 L82 A50 L83 A51 L84 A52 L85 A53 L90 L94 | L0 L84 L88 L90 | L0 L84 L88 L92 | L0 L84 L92 L94 bodies 3 8
sketch "Sketch4" plane through (117.5136, 0, 0) normal (1, 0, 0) x (0, 0, -1)
  line L0 (-1.3824, 0) -> (94.1216, 0)
  line L1 (94.1216, 0) -> (94.1216, 31.242)
  line L2 (94.1216, 31.242) -> (-1.3824, 31.242)
  line L3 (-1.3824, 31.242) -> (-1.3824, 0)
  circle A0 centre (0, 16.4561) radius 4.2071
  circle A1 centre (0, 19.3519) radius 1.7484
sketch "Sketch5" plane through (0, 0, 7.7324) normal (0, 0, 1) x (1, 0, 0)
  line L0 (3.4676, 0) -> (111.1636, 0)
  line L1 (111.1636, 0) -> (111.1636, 31.242)
  line L2 (111.1636, 31.242) -> (3.4676, 31.242)
  line L3 (3.4676, 31.242) -> (3.4676, 0)
  circle A0 centre (22.5176, 11.176) radius 1.8923
  line L4 (-2.8824, 0) -> (-2.8824, 31.242)
  circle A1 centre (32.6776, 11.176) radius 1.8923
  circle A2 centre (92.1136, 11.176) radius 1.8923
  line L5 (117.5136, 31.242) -> (117.5136, 0)
  circle A3 centre (81.9536, 11.176) radius 1.8923
  line L6 (3.4676, 0) -> (111.1636, 0)
  dimension "d90" = 3.7846
  dimension "d91" = 25.4
  dimension "d93" = 3.7846
  dimension "d94" = 10.16
  dimension "d95" = 3.7846
  dimension "d96" = 25.4
  dimension "d98" = 3.7846
  dimension "d99" = 10.16
  dimension "d119" = 11.176
  dimension "d120" = 11.176
  measures "d90" diameter of A0
  measures "d91" distance of A0.centre L4
  measures "d93" diameter of A1
  measures "d94" distance of A0.centre A1.centre
  measures "d95" diameter of A2
  measures "d96" distance of A2.centre L5
  measures "d98" diameter of A3
  measures "d99" distance of A2.centre A3.centre
  measures "d119" distance of A0.centre L6
  measures "d120" distance of A2.centre L6
draft "Draft1" angle 2.375 neutral plane through (0, 12.954, 0) pull (0, 1, 0) 1 faces at (97.5499, 9.2795, -20.0749) on bodies 3
draft "Draft2" angle 2.375 neutral plane through (0, 12.954, 0) pull (0, 1, 0) 1 faces at (28.3368, 9.2795, -26.255) on bodies 3
draft "Draft3" angle 2.375 neutral plane through (0, 12.954, 0) pull (0, 1, 0) 1 faces at (28.3368, 9.2795, -66.254) on bodies 3
fillet "Fillet1" radius 1.6002 8 edges at (117.5136, 0, -46.3696) (115.6537, 0, -98.6117) (57.3156, 0, -100.4716) (-1.0226, 0, -98.6117) (-2.8824, 0, -46.3696) (-1.0226, 0, 5.8725) (57.3156, 0, 7.7324) (115.6537, 0, 5.8725) on bodies 3
sketch "Sketch6" plane through (0, 0, 0) normal (0, 0, 1) x (1, 0, 0)
hidden bodies 3
